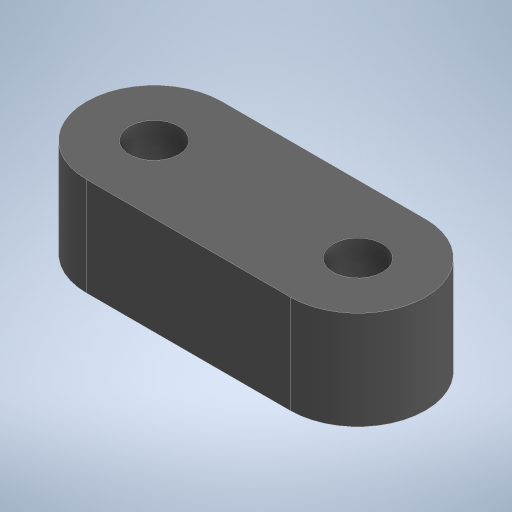
# Autodesk Inventor part: chain_2
Saved by Autodesk Inventor 2024.1 (Build 281209000, 209)
## iProperties
Created: 2025-01-18
Part Number: chain_2
Material: 一般
Document SubType Name: Modeling
Designer: hibik
Density: 1 g/cm^3
Appearance: 既定
Author: hibik
Autodesk Inventor part; units mm, degrees
ref_plane "YZ Plane" through (0, 0, 0) normal (1, 0, 0) x (0, 1, 0)
ref_plane "XZ Plane" through (0, 0, 0) normal (0, 1, 0) x (-1, 0, 0)
ref_plane "XY Plane" through (0, 0, 0) normal (0, 0, 1) x (1, 0, 0)
sketch "スケッチ1" plane through (0, 0, 0) normal (0, 1, 0) x (-1, 0, 0)
  circle A0 centre (0, 0) radius 1
  circle A1 centre (0, 0) radius 2.75
  circle A2 centre (-8.2843, 0) radius 2.75
  circle A3 centre (-8.2843, 0) radius 1
  line L0 (0, -2.75) -> (-8.2843, -2.75)
  line L1 (-8.2843, -2.75) -> (-8.2843, 2.75) construction
  line L2 (-8.2843, 2.75) -> (0, 2.75)
  line L3 (0, 2.75) -> (0, -2.75) construction
  line L4 (-3.55, -2.75) -> (-4.7343, -2.75)
  line L5 (-4.7343, -2.75) -> (-4.7343, 2.75)
  line L6 (-4.7343, 2.75) -> (-3.55, 2.75)
  line L7 (-3.55, 2.75) -> (-3.55, -2.75)
  circle A4 centre (0, 0) radius 3.55 construction
  circle A5 centre (-8.2843, 0) radius 3.55 construction
  circle A6 centre (-4.1421, 10) radius 10
  line L8 (0, 0) -> (-8.2843, 0)
  line L9 (-4.1421, 10) -> (0, 0)
  line L10 (-8.2843, 0) -> (-4.1421, 10)
  point P0 (-3.55, 2.75)
  point P1 (-4.7343, -2.75)
  point P2 (-8.2843, -2.75)
  point P3 (0, 2.75)
  point P4 (-4.1421, 0)
  point P5 (-4.1421, 0)
  point P6 (-4.7343, 0)
  point P7 (-3.55, 0)
  point P8 (-4.7343, 0.0175)
  point P9 (-3.55, 0.0175)
  dimension "d1" = 5.5
  dimension "d0" = 2
  dimension "d7" = 7.1
  dimension "d8" = 7.1
  dimension "d9" = 20
  dimension "d10" = 45
  constraints: 22 end point, 8 coincident, 6 horizontal, 5 centre point, 4 parallel, 3 tangent, 2 midpoint, 2 perpendicular, 2 point on line, 1 equal radius, 1 vertical alignment, 6 other
  measures "d0" diameter of A0
  measures "d7" diameter of A4
  measures "d8" diameter of A5
  measures "d9" diameter of A6
  measures "d10" angle of L10 L9
extrude "押し出し2" add sketch "スケッチ1" along normal blind 4 contours A0 A6 A1 L8 | A0 L9 A1 A6 | L8 A1 A6 A0 | A0 A6 A1 L9 | L8 L7 A6 A1 | A1 L0 L7 L8 | L9 L2 A1 | A1 A6 L7 L2 L9 | L8 A6 L7 | L7 L0 L5 L8 | A6 A3 L8 A2 | A2 L10 A3 A6 | A6 L5 L2 L7 | L8 L5 A6 | L2 L10 A2 | A2 L8 L5 L0 | A6 A2 L10 L2 L5 | L5 L8 A2 A6 | A2 A6 A3 L10 | L8 A3 A6 A2
